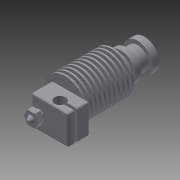
# Autodesk Inventor part: E3Dv6
Saved by Autodesk Inventor 2013 (Build 170138000, 138)
## iProperties
Created: 2014-06-18
Part Number: E3Dv6
Material: Generic
Document SubType Name: Modeling
Designer: employee
Density: 1 g/cm^3
Author: employee
Autodesk Inventor part; units mm, degrees
ref_plane "YZ Plane" through (0, 0, 0) normal (1, 0, 0) x (0, 1, 0)
ref_plane "XZ Plane" through (0, 0, 0) normal (0, 1, 0) x (-1, 0, 0)
ref_plane "XY Plane" through (0, 0, 0) normal (0, 0, 1) x (1, 0, 0)
sketch "Sketch1" plane through (0, 0, 0) normal (0, 0, 1) x (1, 0, 0)
  line L0 (0, 0) -> (-11.15, 0)
  line L1 (-11.15, 0) -> (-11.15, 26)
  line L2 (-11.15, 26) -> (-8, 26)
  line L3 (-8, 26) -> (-8, 33)
  line L4 (-8, 33) -> (-6, 33)
  line L5 (-6, 33) -> (-6, 39)
  line L6 (-6, 39) -> (-8, 39)
  line L7 (-8, 39) -> (-8, 42.7)
  line L8 (-8, 42.7) -> (0, 42.7)
  line L9 (0, 42.7) -> (0, 0)
  dimension "d0" = 6
  dimension "d2" = 8
  dimension "d3" = 11.15
  dimension "d4" = 26
  dimension "d5" = 42.7
  dimension "d6" = 3.7
  dimension "d7" = 6
  constraints: 20 end point, 8 parallel, 1 horizontal, 1 perpendicular, 1 vertical alignment
  measures "d0" distance between parallel lines of L9 L5
  measures "d2" distance of L7.end L8.end
  measures "d3" distance between parallel lines of L1 L9
  measures "d4" distance of L0.end L1.end
  measures "d5" distance between parallel lines of L8 L0
  measures "d6" distance of L6.end L7.end
  measures "d7" distance of L4.end L5.end
revolve "Revolution1" add sketch "Sketch1" angle 360 about axis through (0, 42.7, 0) along (0, -1, 0)
sketch "Sketch2" plane through (0, 0, 0) normal (0, 0, 1) x (1, 0, 0)
  line L0 (11.15, 26) -> (11.15, 0) projected
  line L1 (11.15, 0) -> (-11.15, 0) projected
  line L2 (-11.15, 0) -> (-11.15, 26) projected
  line L3 (-11.15, 26) -> (-8, 26) projected
  line L4 (-8, 26) -> (-8, 33) projected
  line L5 (-8, 33) -> (-6, 33) projected
  line L6 (-6, 33) -> (-6, 39) projected
  line L7 (-6, 39) -> (-8, 39) projected
  line L8 (-8, 39) -> (-8, 42.7) projected
  line L9 (-8, 42.7) -> (8, 42.7) projected
  line L10 (8, 42.7) -> (8, 39) projected
  line L11 (8, 39) -> (6, 39) projected
  line L12 (6, 39) -> (6, 33) projected
  line L13 (6, 33) -> (8, 33) projected
  line L14 (8, 33) -> (8, 26) projected
  line L15 (8, 26) -> (11.15, 26) projected
  line L16 (-11.15, 1) -> (-6, 1)
  line L17 (-6, 1) -> (-6, 2.5)
  line L18 (-6, 2.5) -> (-11.15, 2.5)
  line L19 (-11.15, 2.5) -> (-11.15, 1)
  line L20 (0, -8.54) -> (0, 51.24) projected
  point P0 (0, 0)
  dimension "d9" = 6
  dimension "d10" = 1.5
  dimension "d11" = 1
  constraints: 8 end point, 2 parallel, 1 horizontal, 1 perpendicular, 1 point on line
  measures "d9" distance from line of L17 point (0, 0)
  measures "d10" distance between parallel lines of L18 L16
  measures "d11" distance between parallel lines of L16 L1
revolve "Revolution2" cut sketch "Sketch2" angle 360 about axis through (0, -10, 0) along (0, 1, 0) contours L2 L18 L17 L16
pattern_linear "Rectangular Pattern1" count 12 spacing 2.5 along (0, 1, 0) of "Revolution2"
sketch "Sketch3" plane through (0, 0, 0) normal (0, -1, 0) x (1, 0, 0)
  circle A0 centre (0, 0) radius 11.15 projected
  circle A1 centre (0, 0) radius 1.4
  dimension "d16" = 2.8
  constraints: 1 centre point, 1 coincident
  measures "d16" diameter of A1
extrude "Extrusion1" add sketch "Sketch3" along normal blind 2.1 contours A1
sketch "Sketch4" plane through (0, -2.1, 0) normal (0, -1, 0) x (1, 0, 0)
  circle A0 centre (0, 0) radius 1.4 projected
  line L0 (-4.5, 8) -> (15.5, 8)
  line L1 (15.5, 8) -> (15.5, -8)
  line L2 (15.5, -8) -> (-4.5, -8)
  line L3 (-4.5, -8) -> (-4.5, 8)
  point P0 (-4.5, 0)
  dimension "d20" = 4.5
  dimension "d21" = 16
  dimension "d22" = 20
  constraints: 8 end point, 2 parallel, 1 horizontal, 1 horizontal alignment, 1 midpoint, 1 perpendicular
  measures "d20" distance of A0.centre point (-4.5, 0)
  measures "d21" distance of L2.end L0.start
  measures "d22" distance of L1.end L2.end
extrude "Extrusion2" add sketch "Sketch4" along normal blind 11.5 contours A0 | L0 L1 L2 L3
sketch "Sketch5" plane through (-4.5, -2.1, 8) normal (0, 0, 1) x (1, 0, 0)
  line L0 (0, 0) -> (0, -11.5) projected
  line L1 (20, -11.5) -> (0, -11.5) projected
  line L2 (20, 0) -> (20, -11.5) projected
  circle A0 centre (11.5, -7.5) radius 3
  line L3 (11.5, -6.75) -> (20, -6.75)
  line L4 (20, -6.75) -> (20, -8.25)
  line L5 (20, -8.25) -> (11.5, -8.25)
  line L6 (11.5, -8.25) -> (11.5, -6.75)
  point P0 (4.5, 2.1)
  dimension "d25" = 4
  dimension "d26" = 6
  dimension "d27" = 1.5
  dimension "d28" = 11.5
  constraints: 8 end point, 2 parallel, 1 centre point, 1 coincident, 1 horizontal, 1 midpoint, 1 perpendicular, 1 point on line
  measures "d25" distance from line of A0.centre L1
  measures "d26" diameter of A0
  measures "d27" distance between parallel lines of L3 L5
  measures "d28" distance from line of A0.centre L0
extrude "Extrusion3" cut sketch "Sketch5" against normal through all
sketch "Sketch6" plane through (0, -13.6, 0) normal (0, -1, 0) x (1, 0, 0)
  circle A0 centre (0, 0) radius 2.5
  dimension "d32" = 5
  constraints: 1 centre point, 1 coincident
  measures "d32" diameter of A0
extrude "Extrusion4" add sketch "Sketch6" along normal blind 1.5
fillet "Fillet1" radius 1 14 edges at (5.5, -2.1, 8) (15.5, -5.475, 8) (15.5, -5.475, -8) (15.5, -2.1, 0) (5.5, -2.1, -8) (-4.5, -7.85, -8) (-4.5, -2.1, 0) (-4.5, -7.85, 8) (-4.5, -13.6, 0) (5.5, -13.6, -8) (15.5, -11.975, -8) (15.5, -13.6, 0) (15.5, -11.975, 8) (5.5, -13.6, 8)
sketch "Sketch7" plane through (0, -15.1, 0) normal (0, -1, 0) x (1, 0, 0)
  circle A0 centre (0, 0) radius 2.5 projected
  line L0 (2.0207, 3.5) -> (4.0415, 0)
  line L1 (4.0415, 0) -> (2.0207, -3.5)
  line L2 (2.0207, -3.5) -> (-2.0207, -3.5)
  line L3 (-2.0207, -3.5) -> (-4.0415, 0)
  line L4 (-4.0415, 0) -> (-2.0207, 3.5)
  line L5 (-2.0207, 3.5) -> (2.0207, 3.5)
  dimension "d36" = 7
  constraints: 12 end point, 1 coincident, 1 horizontal, 13 other
  measures "d36" distance between parallel lines of L2 L5
extrude "Extrusion5" add sketch "Sketch7" along normal blind 3 contours A0 | L0 L1 L2 L3 L4 L5
sketch "Sketch8" plane through (0, 0, 0) normal (0, 0, 1) x (1, 0, 0)
  line L0 (6, 2.5) -> (6, 1) projected
  line L1 (6, 1) -> (11.15, 1) projected
  line L2 (11.15, 1) -> (11.15, 0) projected
  line L3 (11.15, 0) -> (1.4, 0) projected
  line L4 (1.4, 0) -> (1.4, -2.1) projected
  line L5 (1.4, -2.1) -> (14.5, -2.1) projected
  arc A0 (15.5, -3.1) -> (14.5, -2.1) centre (14.5, -3.1) ccw projected
  line L6 (15.5, -3.1) -> (15.5, -8.85) projected
  line L7 (15.5, -8.85) -> (9.9047, -8.85) projected
  arc A1 (9.9047, -8.85) -> (9.9047, -10.35) centre (7, -9.6) ccw projected
  line L8 (9.9047, -10.35) -> (15.5, -10.35) projected
  line L9 (15.5, -10.35) -> (15.5, -12.6) projected
  arc A2 (14.5, -13.6) -> (15.5, -12.6) centre (14.5, -12.6) ccw projected
  line L10 (14.5, -13.6) -> (2.5, -13.6) projected
  line L11 (2.5, -13.6) -> (2.5, -15.1) projected
  line L12 (2.5, -15.1) -> (4.0415, -15.1) projected
  line L13 (4.0415, -15.1) -> (4.0415, -18.1) projected
  line L14 (4.0415, -18.1) -> (-4.0415, -18.1) projected
  line L15 (-4.0415, -18.1) -> (-4.0415, -15.1) projected
  line L16 (-4.0415, -15.1) -> (-2.5, -15.1) projected
  line L17 (-2.5, -15.1) -> (-2.5, -13.6) projected
  line L18 (-2.5, -13.6) -> (-3.5, -13.6) projected
  arc A3 (-4.5, -12.6) -> (-3.5, -13.6) centre (-3.5, -12.6) ccw projected
  line L19 (-4.5, -12.6) -> (-4.5, -3.1) projected
  arc A4 (-3.5, -2.1) -> (-4.5, -3.1) centre (-3.5, -3.1) ccw projected
  line L20 (-3.5, -2.1) -> (-1.4, -2.1) projected
  line L21 (-1.4, -2.1) -> (-1.4, 0) projected
  line L22 (-1.4, 0) -> (-11.15, 0) projected
  line L23 (-11.15, 0) -> (-11.15, 1) projected
  line L24 (-11.15, 1) -> (-6, 1) projected
  line L25 (-6, 1) -> (-6, 2.5) projected
  line L26 (-6, 2.5) -> (-11.15, 2.5) projected
  line L27 (-11.15, 2.5) -> (-11.15, 3.5) projected
  line L28 (-11.15, 3.5) -> (-6, 3.5) projected
  line L29 (-6, 3.5) -> (-6, 5) projected
  line L30 (-6, 5) -> (-11.15, 5) projected
  line L31 (-11.15, 5) -> (-11.15, 6) projected
  line L32 (-11.15, 6) -> (-6, 6) projected
  line L33 (-6, 6) -> (-6, 7.5) projected
  line L34 (-6, 7.5) -> (-11.15, 7.5) projected
  line L35 (-11.15, 7.5) -> (-11.15, 8.5) projected
  line L36 (-11.15, 8.5) -> (-6, 8.5) projected
  line L37 (-6, 8.5) -> (-6, 10) projected
  line L38 (-6, 10) -> (-11.15, 10) projected
  line L39 (-11.15, 10) -> (-11.15, 11) projected
  line L40 (-11.15, 11) -> (-6, 11) projected
  line L41 (-6, 11) -> (-6, 12.5) projected
  line L42 (-6, 12.5) -> (-11.15, 12.5) projected
  line L43 (-11.15, 12.5) -> (-11.15, 13.5) projected
  line L44 (-11.15, 13.5) -> (-6, 13.5) projected
  line L45 (-6, 13.5) -> (-6, 15) projected
  line L46 (-6, 15) -> (-11.15, 15) projected
  line L47 (-11.15, 15) -> (-11.15, 16) projected
  line L48 (-11.15, 16) -> (-6, 16) projected
  line L49 (-6, 16) -> (-6, 17.5) projected
  line L50 (-6, 17.5) -> (-11.15, 17.5) projected
  line L51 (-11.15, 17.5) -> (-11.15, 18.5) projected
  line L52 (-11.15, 18.5) -> (-6, 18.5) projected
  line L53 (-6, 18.5) -> (-6, 20) projected
  line L54 (-6, 20) -> (-11.15, 20) projected
  line L55 (-11.15, 20) -> (-11.15, 21) projected
  line L56 (-11.15, 21) -> (-6, 21) projected
  line L57 (-6, 21) -> (-6, 22.5) projected
  line L58 (-6, 22.5) -> (-11.15, 22.5) projected
  line L59 (-11.15, 22.5) -> (-11.15, 23.5) projected
  line L60 (-11.15, 23.5) -> (-6, 23.5) projected
  line L61 (-6, 23.5) -> (-6, 25) projected
  line L62 (-6, 25) -> (-11.15, 25) projected
  line L63 (-11.15, 25) -> (-11.15, 26) projected
  line L64 (-11.15, 26) -> (-6, 26) projected
  line L65 (-6, 26) -> (-6, 27.5) projected
  line L66 (-6, 27.5) -> (-8, 27.5) projected
  line L67 (-8, 27.5) -> (-8, 28.5) projected
  line L68 (-8, 28.5) -> (-6, 28.5) projected
  line L69 (-6, 28.5) -> (-6, 30) projected
  line L70 (-6, 30) -> (-8, 30) projected
  line L71 (-8, 30) -> (-8, 33) projected
  line L72 (-8, 33) -> (-6, 33) projected
  line L73 (-6, 33) -> (-6, 39) projected
  line L74 (-6, 39) -> (-8, 39) projected
  line L75 (-8, 39) -> (-8, 42.7) projected
  line L76 (-8, 42.7) -> (8, 42.7) projected
  line L77 (8, 42.7) -> (8, 39) projected
  line L78 (8, 39) -> (6, 39) projected
  line L79 (6, 39) -> (6, 33) projected
  line L80 (6, 33) -> (8, 33) projected
  line L81 (8, 33) -> (8, 30) projected
  line L82 (8, 30) -> (6, 30) projected
  line L83 (6, 30) -> (6, 28.5) projected
  line L84 (6, 28.5) -> (8, 28.5) projected
  line L85 (8, 28.5) -> (8, 27.5) projected
  line L86 (8, 27.5) -> (6, 27.5) projected
  line L87 (6, 27.5) -> (6, 26) projected
  line L88 (6, 26) -> (11.15, 26) projected
  line L89 (11.15, 26) -> (11.15, 25) projected
  line L90 (11.15, 25) -> (6, 25) projected
  line L91 (6, 25) -> (6, 23.5) projected
  line L92 (6, 23.5) -> (11.15, 23.5) projected
  line L93 (11.15, 23.5) -> (11.15, 22.5) projected
  line L94 (11.15, 22.5) -> (6, 22.5) projected
  line L95 (6, 22.5) -> (6, 21) projected
  line L96 (6, 21) -> (11.15, 21) projected
  line L97 (11.15, 21) -> (11.15, 20) projected
  line L98 (11.15, 20) -> (6, 20) projected
  line L99 (6, 20) -> (6, 18.5) projected
  line L100 (6, 18.5) -> (11.15, 18.5) projected
  line L101 (11.15, 18.5) -> (11.15, 17.5) projected
  line L102 (11.15, 17.5) -> (6, 17.5) projected
  line L103 (6, 17.5) -> (6, 16) projected
  line L104 (6, 16) -> (11.15, 16) projected
  line L105 (11.15, 16) -> (11.15, 15) projected
  line L106 (11.15, 15) -> (6, 15) projected
  line L107 (6, 15) -> (6, 13.5) projected
  line L108 (6, 13.5) -> (11.15, 13.5) projected
  line L109 (11.15, 13.5) -> (11.15, 12.5) projected
  line L110 (11.15, 12.5) -> (6, 12.5) projected
  line L111 (6, 12.5) -> (6, 11) projected
  line L112 (6, 11) -> (11.15, 11) projected
  line L113 (11.15, 11) -> (11.15, 10) projected
  line L114 (11.15, 10) -> (6, 10) projected
  line L115 (6, 10) -> (6, 8.5) projected
  line L116 (6, 8.5) -> (11.15, 8.5) projected
  line L117 (11.15, 8.5) -> (11.15, 7.5) projected
  line L118 (11.15, 7.5) -> (6, 7.5) projected
  line L119 (6, 7.5) -> (6, 6) projected
  line L120 (6, 6) -> (11.15, 6) projected
  line L121 (11.15, 6) -> (11.15, 5) projected
  line L122 (11.15, 5) -> (6, 5) projected
  line L123 (6, 5) -> (6, 3.5) projected
  line L124 (6, 3.5) -> (11.15, 3.5) projected
  line L125 (11.15, 3.5) -> (11.15, 2.5) projected
  line L126 (11.15, 2.5) -> (6, 2.5) projected
  line L127 (0, -18.1) -> (0, -20.1)
  line L128 (0, -20.1) -> (-0.5, -20.1)
  line L129 (-0.5, -20.1) -> (-1.9004, -18.1)
  point P0 (0, 0)
  dimension "d39" = 125
  dimension "d41" = 0.5
  dimension "d42" = 2
  constraints: 6 end point, 2 perpendicular, 1 midpoint, 1 point on line
  measures "d39" angle of L14 L129
  measures "d41" distance of L127.end L128.end
  measures "d42" distance of L127.start L127.end
revolve "Revolution3" add sketch "Sketch8" angle 360 about axis through (0, -18.1, 0) along (0, -1, 0) contours L127 L128 L129 L14
body "Solid1"
